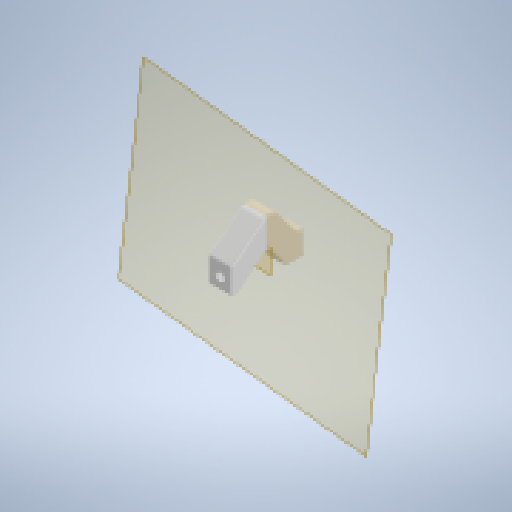
# Autodesk Inventor part: Neck
Saved by Autodesk Inventor 2025.2 (Build 292293000, 293)
## iProperties
Created: 2025-02-23
Part Number: Neck
Material: Generic
Document SubType Name: Modeling
Designer: andre
Density: 1 g/cm^3
Appearance: Default
Author: andre
Autodesk Inventor part; units mm, degrees
ref_plane "YZ Plane" through (0, 0, 0) normal (1, 0, 0) x (0, 1, 0)
ref_plane "XZ Plane" through (0, 0, 0) normal (0, 1, 0) x (-1, 0, 0)
ref_plane "XY Plane" through (0, 0, 0) normal (0, 0, 1) x (1, 0, 0)
sketch "Sketch3" plane through (0, 0, 0) normal (1, 0, 0) x (0, 1, 0)
  line L0 (-37, 0) -> (37, 0) construction
  line L1 (0, 5) -> (11.995218, 14.131243) construction
  line L2 (3.028543, 1.021567) -> (15.023761, 10.152811)
  line L3 (8.966674, 18.109676) -> (-3.028543, 8.978433)
  arc A0 (-3.028543, 8.978433) -> (3.028543, 1.021567) centre (0, 5) ccw
  arc A1 (15.023761, 10.152811) -> (8.966674, 18.109676) centre (11.995218, 14.131243) ccw
  line L4 (0, -9.617943) -> (0, 43.658825) construction
  line L5 (11.995218, 14.131243) -> (0, 29.017329) construction
  line L6 (15.888521, 17.26847) -> (3.893303, 32.154555)
  line L7 (-3.893303, 25.880102) -> (8.101914, 10.994017)
  arc A2 (8.101914, 10.994017) -> (15.888521, 17.26847) centre (11.995218, 14.131243) ccw
  arc A3 (3.893303, 32.154555) -> (-3.893303, 25.880102) centre (0, 29.017329) ccw
  point P0 (5.997609, 9.565622)
  point P1 (5.997609, 21.574286)
  point P2 (4.876845, 14.996333)
  dimension "d8" = 10
  dimension "d9" = 10
  constraints: 16 end point, 9 tangent, 8 point on circle, 4 centre point, 2 midpoint, 2 parallel, 2 point on line
  measures "d8" diameter of A1
  measures "d9" diameter of A3
extrude "Extrusion3" add sketch "Sketch3" along normal mid plane 10
sketch "Sketch4" plane through (0, 0, 0) normal (0, 0, 1) x (1, 0, 0)
  line L0 (-5, -5) -> (5, -5) projected
  line L1 (5, 5) -> (-5, 5)
  line L2 (-5, 5) -> (-5, -5)
  line L3 (-5, -5) -> (5, -5)
  line L4 (5, -5) -> (5, 5)
  line L5 (5, 5) -> (-5, -5) construction
  line L6 (-5, 5) -> (5, -5) construction
  point P0 (0, 0)
  constraints: 12 end point, 2 midpoint, 2 parallel, 1 horizontal, 1 perpendicular
extrude "Extrusion4" add sketch "Sketch4" along normal up to surface round surface about axis through (0, 0, 5) along (1, 0, 0) radius 5 far side no
fillet "Fillet1" radius 2 2 edges at (0, 5, 2.5223) (0, 4.8768, 14.9963)
fillet "Fillet2" radius 0.5 4 edges at (5, 0, 0) (0, 5, 0) (-5, 0, 0) (0, -5, 0)
ref_plane "Work Plane1" through (0, 0, 15.5) normal (0, 0, 1) x (0.9928144, -0.1196643, 0)
sketch "Sketch5" plane through (0, 0, 15.5) normal (0, 0, 1) x (0.9928144, -0.1196643, 0)
  circle A0 centre (0, 0) radius 2.6
  dimension "d16" = 5.2
  constraints: 1 centre point, 1 coincident
  measures "d16" diameter of A0
extrude "Extrusion5" cut sketch "Sketch5" against normal blind 13
fillet "Fillet3" radius 0.5 1 edges at (-2.5813, 0.3111, 11.5207)
fillet "Fillet4" radius 0.5 1 edges at (-2.5813, 0.3111, 2.5)
sketch "Sketch6" plane through (0, 0, 2.5) normal (0, 0, 1) x (1, 0, 0)
  circle A0 centre (0, 0) radius 1.45 projected
  point P0 (0, 0)
extrude "Extrusion6" cut sketch "Sketch6" against normal up to next
fillet "Fillet5" radius 0.5 2 edges at (-1.45, 0, 0) (-1.45, 0, 2.5)
sketch "Sketch7" plane through (5, 0, 0) normal (1, 0, 0) x (0, 0, -1)
  line L0 (-30.011825, 6.312681) -> (-30.011825, -2.937319) construction
  line L1 (-0.5, 5) -> (-0.5, -5) construction
  line L2 (-0.5, 5) -> (-1.531248, 5) construction
  arc A0 (-3.122621, 5.788583) -> (-1.531248, 5) centre (-1.531248, 7) ccw construction
  line L3 (-3.122621, 5.788583) -> (-10.152811, 15.023761) construction
  arc A1 (-10.152811, 15.023761) -> (-17.26847, 15.888521) centre (-14.131243, 11.995218) ccw construction
  line L4 (-17.26847, 15.888521) -> (-32.154555, 3.893303)
  arc A2 (-32.154555, 3.893303) -> (-25.880102, -3.893303) centre (-29.017329, 0) ccw construction
  line L5 (-25.880102, -3.893303) -> (-16.597259, 3.586818) construction
  arc A3 (-13.750996, 3.240914) -> (-16.597259, 3.586818) centre (-15.342369, 2.029496) ccw construction
  line L6 (-13.750996, 3.240914) -> (-8.978433, -3.028543) construction
  arc A4 (-8.978433, -3.028543) -> (-5, -5) centre (-5, 0) ccw construction
  line L7 (-0.5, -5) -> (-5, -5) construction
  arc A5 (-32.154555, 3.893303) -> (-25.880102, -3.893303) centre (-29.017329, 0) ccw
  line L8 (-30.011825, -4.9001) -> (-30.011825, 5.619917)
  point P0 (0, 0)
  constraints: 2 end point, 2 point on line, 1 point on circle
extrude "Extrusion7" cut sketch "Sketch7" against normal up to next
fillet "Fillet6" radius 1 1 edges at (0, -4.9001, 30.0118)
fillet "Fillet7" radius 1 1 edges at (0, 5.6199, 30.0118)
sketch "Sketch8" plane through (-5, -3.999996, 30.011825) normal (0, 0, 1) x (1, 0, 0)
  circle A0 centre (5, 3.999996) radius 1.45
  point P0 (5, 3.999996)
extrude "Extrusion8" cut sketch "Sketch8" against normal up to next
ref_plane "Work Plane2" through (-5, -3.999996, 14.511825) normal (0, 0, 1) x (1, 0, 0)
sketch "Sketch9" plane through (-5, -3.999996, 14.511825) normal (0, 0, 1) x (1, 0, 0)
  arc A0 (6.238516, 1.713935) -> (3.761484, 1.713935) centre (5, 3.999996) ccw
  spline S0 degree 9 poles (6.238517, 1.713934) (6.002489, 1.586044) (5.744444, 1.481626) (5.462931, 1.404774) (5.162222, 1.35771) (4.836002, 1.357917) (4.53569, 1.405118) (4.254607, 1.482001) (3.997049, 1.586294) (3.761483, 1.713934) knots 0 0 0 0 0 0 0 0 0 0 1 1 1 1 1 1 1 1 1 1 weights 1.05917158 1.06320672 1.06703547 1.0702415 1.07252874 1.07251731 1.0702267 1.06702149 1.0631988 1.05917158
  circle A1 centre (5, 3.999996) radius 2.6
  arc A2 (6.550997, 1.137156) -> (3.449003, 1.137156) centre (5, 3.999996) ccw
  spline S1 degree 4 poles (6.551029, 1.137172) (5.84085, 0.752154) (5, 0.602104) (4.15915, 0.752154) (3.44897, 1.137172) knots 0 0 0 0 0 1 1 1 1 1
  constraints: 2 horizontal alignment, 2 point on circle, 1 centre point, 1 concentric, 2 other
extrude "Extrusion9" cut sketch "Sketch9" along normal blind 12.5 contours S0 A0 | S1 A2
fillet "Fillet8" radius 0.5 2 edges at (0, -3.256, 25.0892) (0, 3.256, 17.0078)
fillet "Fillet9" radius 0.5 4 edges at (0, -3.256, 27.0118) (0, 3.256, 27.0118) (-1.45, 0, 27.0118) (-1.45, 0, 30.0118)
fillet "Fillet10" radius 1 32 edges at (-5, 10.4062, 6.6377) (-5, 5.208, 2.4193) (-5, 5, 1.0156) (-4.8536, 4.8536, 0.1464) (-5, 10.9043, 23.4539) (-5, 5.5731, 29.9139) (-5, 0.5707, 30.0118) (-5, -4.7076, 29.7184) (-5, -4.7141, 27.3507) (-5, -0.1532, 21.2387) (-5, 4.0149, 15.1011) (-5, 0.1062, 11.3647) (-5, -4.4801, 7.2201) (-5, -5, 2.75) (-4.8536, -4.8536, 0.1464) (-5, 16.9587, 13.528) (5, 10.9043, 23.4539) (5, 5.5731, 29.9139) (5, 0.5707, 30.0118) (5, -4.7076, 29.7184) (5, -4.7141, 27.3507) (5, -0.1532, 21.2387) (5, 4.0149, 15.1011) (5, 0.1062, 11.3647) (5, -4.4801, 7.2201) (5, -5, 2.75) (4.8536, -4.8536, 0.1464) (5, 10.4062, 6.6377) (5, 5.208, 2.4193) (5, 5, 1.0156) (4.8536, 4.8536, 0.1464) (5, 16.9587, 13.528)
equation "\"d10\" = d8"
body "Solid2"
